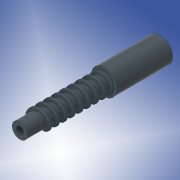
# Autodesk Inventor part: BA014
Saved by Autodesk Inventor 2017 SP1 (Build 210196100, 196)
## iProperties
Created: 2017-06-28
Part Number: BA014
Material: ABS Plastic
Document SubType Name: Modeling
Designer: zallen
Density: 1.06 g/cm^3
Appearance: CR Dark Blue
Author: zallen
Autodesk Inventor part; units mm, degrees
ref_plane "YZ Plane" through (0, 0, 0) normal (1, 0, 0) x (0, 1, 0)
ref_plane "XZ Plane" through (0, 0, 0) normal (0, 1, 0) x (-1, 0, 0)
ref_plane "XY Plane" through (0, 0, 0) normal (0, 0, 1) x (1, 0, 0)
sketch "Sketch5" plane through (0, 0, 0) normal (0, 0, 1) x (1, 0, 0)
  circle A0 centre (0, 0) radius 5.5
  dimension "d13" = 11
  constraints: 1 centre point, 1 coincident
  measures "d13" diameter of A0
extrude "Extrusion2" add sketch "Sketch5" along normal blind 100
sketch "Sketch7" plane through (0, 0, 100) normal (0, 0, 1) x (1, 0, 0)
  circle A0 centre (0, 0) radius 2.75
  dimension "d29" = 5.5
  constraints: 1 centre point, 1 coincident
  measures "d29" diameter of A0
extrude "Extrusion3" cut sketch "Sketch7" against normal through all
sketch "Sketch6" plane through (0, 0, 0) normal (0, 1, 0) x (-1, 0, 0)
  line L0 (5.5, 100) -> (-5.5, 100) projected
  line L1 (5.5, 0) -> (5.5, 100) projected
  line L2 (5.5, 89) -> (7.5, 89)
  line L3 (7.5, 89) -> (7.5, 87)
  line L4 (7.5, 87) -> (5.5, 87)
  line L5 (5.5, 89) -> (5.5, 87)
  line L6 (0, 100) -> (0, 0)
  point P0 (7.5, 88)
  dimension "d17" = 2
  dimension "d18" = 2
  dimension "d20" = 11
  constraints: 10 end point, 3 perpendicular, 2 coincident, 2 midpoint, 2 vertical, 1 point on line
  measures "d17" distance of L2.start L2.end
  measures "d18" distance of L2.end L3.end
  measures "d20" distance between parallel lines of L0 L2
coil "Coil2" sketch "Sketch6" operation add axis through (0, 0, 100) along (0, 0, -1) pitch 5.6 turns 10 hand right
chamfer "Chamfer1" distance 0.5 angle 45 40 edges at (0, 7.5, 87.6) (0, 7.5, 82) (0, -7.5, 84.8) (0, -7.5, 79.2) (0, 7.5, 76.4) (0, -7.5, 73.6) (0, 7.5, 70.8) (0, -7.5, 68) (0, 7.5, 65.2) (0, -7.5, 34.4) (0, -7.5, 62.4) (0, 7.5, 59.6) (0, 7.5, 37.2) (0, -7.5, 40) (0, -7.5, 56.8) (0, 7.5, 54) (0, 7.5, 42.8) (0, -7.5, 45.6) (0, -7.5, 51.2) (0, 7.5, 48.4) (0, 7.5, 85.6) (0, -7.5, 82.8) (0, 7.5, 80) (0, -7.5, 77.2) (0, 7.5, 74.4) (0, -7.5, 71.6) (0, 7.5, 68.8) (0, -7.5, 32.4) (0, -7.5, 38) (0, 7.5, 35.2) (0, -7.5, 66) (0, 7.5, 63.2) (0, -7.5, 43.6) (0, 7.5, 40.8) (0, -7.5, 60.4) (0, 7.5, 57.6) (0, -7.5, 49.2) (0, 7.5, 46.4) (0, -7.5, 54.8) (0, 7.5, 52)
sketch "Sketch9" plane through (0, 0, 0) normal (0, 0, -1) x (-1, 0, 0)
  circle A0 centre (0, 0) radius 2.75 projected
  circle A1 centre (0, 0) radius 5.5 projected
  circle A2 centre (0, 0) radius 9
  dimension "d39" = 18
  constraints: 1 centre point, 1 coincident
  measures "d39" diameter of A2
extrude "Extrusion5" add sketch "Sketch9" against normal blind 40 contours A2
sketch "Sketch8" plane through (0, 0, 0) normal (1, 0, 0) x (0, 1, 0)
  circle A0 centre (0, 10) radius 1.5
  point P0 (0, 0)
  dimension "d35" = 3
  dimension "d36" = 10
  constraints: 1 centre point, 1 vertical alignment
  measures "d35" diameter of A0
  measures "d36" distance of point (0, 0) A0.centre
extrude "Extrusion4" cut sketch "Sketch8" against normal through all
body "Solid2"
